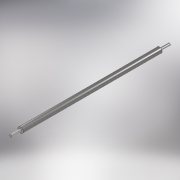
# Autodesk Inventor part: Fuso
Saved by Autodesk Inventor 2022 (Build 260153000, 153)
## iProperties
Created: 2023-03-17
Part Number: Fuso
Material: Aço galvanizado
Document SubType Name: Sheet Metal
Designer: Mateus
Density: 7.85 g/cm^3
Sheet Metal Rule: Padrão_mm
Appearance: Galvanizado
Author: Mateus
Autodesk Inventor part; units mm, degrees
ref_plane "YZ Plane" through (0, 0, 0) normal (1, 0, 0) x (0, 1, 0)
ref_plane "XZ Plane" through (0, 0, 0) normal (0, 1, 0) x (-1, 0, 0)
ref_plane "XY Plane" through (0, 0, 0) normal (0, 0, 1) x (1, 0, 0)
sketch "Esboço1" plane through (0, 0, 0) normal (0, 1, 0) x (-1, 0, 0)
  line L0 (0, 0) -> (3, 0)
  line L1 (3, 0) -> (3, -25)
  line L2 (3, -25) -> (7, -25)
  line L3 (7, -25) -> (7, -375)
  line L4 (7, -375) -> (3, -375)
  line L5 (3, -375) -> (3, -400)
  line L6 (3, -400) -> (0, -400)
  line L7 (0, -400) -> (0, 0)
  dimension "d0" = 3
  dimension "d1" = 25
  dimension "d2" = 4
  dimension "d3" = 350
  dimension "d4" = 4
  dimension "d5" = 25
  constraints: 16 end point, 6 perpendicular, 2 horizontal
  measures "d0" distance of L0.start L0.end
  measures "d1" distance of L0.end L1.end
  measures "d2" distance of L1.end L2.end
  measures "d3" distance of L2.end L3.end
  measures "d4" distance of L3.end L4.end
  measures "d5" distance of L4.end L5.end
revolve "Revolução1" add sketch "Esboço1" angle 360 about axis through (0, 0, -400) along (0, 0, 1)
thread "Rosca1" size "M14x2" class "6g" standard "ANSI Metric M Profile" full length
equation "\"Raio_vergadura\" = Espessura"
equation "\"Largura_alívio_de_vergadura\" = Espessura"
equation "\"Profundidade_alívio_de_vergadura\" = 0.5 * Espessura"
equation "\"Tamanho_alívio_de_dobra\" = 4 * Espessura"
equation "\"Remanescente_mínimo\" = 2 * Espessura"
equation "\"Raiodetransição\" = Raio_vergadura"
equation "\"Tamanho_de_raio_de_Jacobi\" = Raio_vergadura"
equation "\"TamanhoFolga\" = Espessura"
equation "\"Espessura\" = 0.5"
